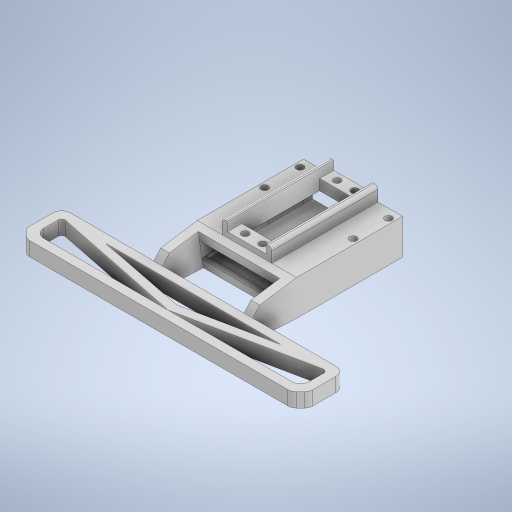
# Autodesk Inventor part: Pieza2
Saved by Autodesk Inventor 2024.3 (Build 283343000, 343)
## iProperties
Created: 2025-01-30
Part Number: Pieza2
Material: Genérico
Document SubType Name: Modeling
Designer: Jorge
Density: 1 g/cm^3
Appearance: Valor por defecto
Author: Jorge
Autodesk Inventor part; units mm, degrees
sketch "Boceto1" plane through (0, 0, 0) normal (0, 1, 0) x (-1, 0, 0)
  line L0 (0, 0) -> (0, -60)
  line L1 (0, 0) -> (30, 0)
  line L2 (0, -60) -> (30, -60)
  line L3 (30, -60) -> (30, 0)
  line L4 (0, 0) -> (-26, 0)
  line L5 (-26, 0) -> (-26, -60)
  line L6 (-26, -60) -> (0, -60)
  dimension "d0" = 60
  dimension "d1" = 30
  dimension "d2" = 30
  dimension "d3" = 26
  constraints: 14 end point, 3 horizontal, 1 collinear, 1 perpendicular, 1 vertical
  measures "d0" distance of L0.start L0.end
  measures "d1" distance of L0.start L1.end
  measures "d2" distance of L0.end L2.end
  measures "d3" distance of L0.start L4.end
extrude "Extrusión1" add sketch "Boceto1" along normal blind 20
sketch "Boceto2" plane through (-30, 0, 0) normal (0, 0, 1) x (1, 0, 0)
  line L0 (56, 0) -> (0, 0) construction
  line L1 (28, 0) -> (28, 20) construction
  line L2 (56, 20) -> (0, 20) construction
  line L3 (0, 0) -> (0, 20) construction
  line L4 (0, 10) -> (5, 10) construction
  line L5 (56, 0) -> (56, 20) construction
  line L6 (56, 10) -> (51, 10) construction
  line L7 (28, 20) -> (28, 17) construction
  line L8 (28, 17) -> (51, 17)
  line L9 (51, 17) -> (51, 10)
  line L10 (28, 17) -> (5, 17)
  line L11 (5, 17) -> (5, 10)
  line L12 (28, 0) -> (28, 3) construction
  line L13 (28, 3) -> (5, 3)
  line L14 (5, 3) -> (5, 10)
  line L15 (28, 3) -> (51, 3)
  line L16 (51, 3) -> (51, 10)
  point P0 (30, 0)
  dimension "d8" = 3
  dimension "d9" = 3
  constraints: 26 end point, 5 perpendicular, 4 midpoint, 4 point on line, 2 horizontal, 1 collinear
  measures "d8" distance of L1.end L7.end
  measures "d9" distance of L1.start L12.end
extrude "Extrusión2" cut sketch "Boceto2" against normal through all
sketch "Boceto3" plane through (0, 20, 0) normal (0, 1, 0) x (1, 0, 0)
  line L0 (21, 60) -> (-25, 60) projected
  line L1 (-2, 60) -> (-2, 0)
  line L2 (-25, 0) -> (21, 0) projected
  line L3 (-2, 0) -> (12, 0) construction
  line L4 (-2, 0) -> (-16, 0) construction
  line L5 (-16, 0) -> (-16, 60) construction
  line L6 (-16, 60) -> (12, 60)
  line L7 (12, 60) -> (12, 0)
  line L8 (12, 0) -> (-16, 0)
  line L9 (-16, 0) -> (-16, 60)
  point P0 (0, 0)
  point P1 (12, 60)
  dimension "d12" = 14
  dimension "d13" = 14
  constraints: 16 end point, 3 point on line, 2 midpoint, 2 parallel, 2 perpendicular, 1 horizontal
  measures "d12" distance of L1.end L3.end
  measures "d13" distance of L1.end L4.end
extrude "Extrusión3" add sketch "Boceto3" along normal blind 8
sketch "Boceto4" plane through (0, 28, 0) normal (0, 1, 0) x (1, 0, 0)
  line L0 (12, 0) -> (26, 0) construction
  line L1 (12, 0) -> (9, 0) construction
  line L2 (9, 0) -> (9, 60)
  line L3 (26, 60) -> (-30, 60) projected
  line L4 (-16, 0) -> (-16, 60) projected
  line L5 (-16, 0) -> (-13, 0)
  line L6 (-30, 0) -> (26, 0) projected
  line L7 (-13, 0) -> (-13, 60)
  line L8 (-2, 0) -> (-2, 8) construction
  line L9 (-13, 8) -> (9, 8)
  line L10 (-2, 60) -> (-2, 52) construction
  line L11 (-13, 52) -> (9, 52)
  line L12 (9, 56) -> (5, 56) construction
  line L13 (-13, 30) -> (9, 30) construction
  line L14 (5, 56) -> (3, 56) construction
  circle A0 centre (3, 56) radius 2
  circle A1 centre (-7, 56) radius 2
  circle A2 centre (3, 4) radius 2
  circle A3 centre (-7, 4) radius 2
  point P0 (0, 0)
  dimension "d16" = 3
  dimension "d17" = 3
  dimension "d18" = 8
  dimension "d19" = 8
  dimension "d20" = 4
  dimension "d21" = 2
  constraints: 22 end point, 8 point on line, 4 midpoint, 3 centre point, 3 horizontal, 3 perpendicular, 3 symmetric about line, 3 vertical, 1 coincident, 1 horizontal alignment, 5 other
  measures "d16" distance of L0.start L1.end
  measures "d17" distance of L4.start L5.end
  measures "d18" distance of L8.start L8.end
  measures "d19" distance of L10.start L10.end
  measures "d20" distance of L12.start L12.end
  measures "d21" distance of L12.end L14.end
extrude "Extrusión4" cut sketch "Boceto4" against normal blind 15 contours L9 L7 L11 L2
extrude "Extrusión5" cut sketch "Boceto4" against normal blind 15 contours A0 | A1 | A2 | A3
extrude "Extrusión6" cut sketch "Boceto4" against normal blind 5 contours L6 L7 L9 L2 | L11 L7 L3 L2
fillet "Empalme1" radius 2 2 edges at (-16, 28, -30) (12, 28, -30)
ref_plane "Plano de trabajo1" through (-2, 0, 0) normal (1, 0, 0) x (0, 1, 0)
sketch "Boceto6" plane through (-2, 0, 0) normal (1, 0, 0) x (0, 1, 0)
  line L0 (0, 0) -> (20, 0) projected
  line L1 (28, 0) -> (23, 0) projected
  line L2 (28, 0) -> (0, 0)
  line L3 (20, 0) -> (16.2743, 24.7208)
  line L4 (16.2743, 24.7208) -> (1.2743, 24.7208)
  line L5 (1.2743, 24.7208) -> (0, 0)
  line L6 (0, 0) -> (20, 0)
  dimension "d32" = 25
  dimension "d33" = 15
  constraints: 10 end point, 2 horizontal, 1 collinear
  measures "d32" distance of L0.end L3.end
  measures "d33" distance of L3.end L4.end
extrude "Extrusión7" add sketch "Boceto6" along normal mid plane 56
sketch "Boceto7" plane through (-30, 16.2743, 24.7208) normal (0, 0.9888, 0.149) x (1, 0, 0)
  line L0 (56, -2.2354) -> (56, 22.0194) construction
  line L1 (56, 9.892) -> (51, 9.892) construction
  line L2 (0, 22.0194) -> (0, -2.2354) construction
  line L3 (0, 11.3809) -> (5, 11.3809) construction
  line L4 (39, 25.4471) -> (17, 25.4471) construction
  line L5 (28, 25.4471) -> (28, 20.4471) construction
  line L6 (0, 0) -> (56, 0) projected
  line L7 (5, 0) -> (51, 0)
  line L8 (51, 0) -> (51, 20.4471)
  line L9 (51, 20.4471) -> (5, 20.4471)
  line L10 (5, 20.4471) -> (5, 0)
  line L11 (5, 0) -> (5, -22.0119)
  line L12 (5, -22.0119) -> (51, -22.0119)
  line L13 (51, -22.0119) -> (51, 0)
  point P0 (30, 22.0194)
  dimension "d36" = 5
  dimension "d38" = 5
  dimension "d39" = 5
  constraints: 20 end point, 3 horizontal, 2 midpoint, 2 parallel, 2 perpendicular, 2 point on line, 2 vertical, 1 collinear
  measures "d36" distance of L1.start L1.end
  measures "d38" distance of L3.start L3.end
  measures "d39" distance of L5.start L5.end
extrude "Extrusión8" cut sketch "Boceto7" against normal blind 56
ref_plane "Plano de trabajo2" through (26, 0, 24.73) normal (0, 0, -1) x (-1, 0, 0)
sketch "Boceto8" plane through (26, 0, 24.73) normal (0, 0, -1) x (-1, 0, 0)
  line L0 (17, 23) -> (39, 23) construction
  line L1 (28, 23) -> (28, 0) construction
  line L2 (56, 0) -> (0, 0) construction
  line L3 (28, 8.5182) -> (108, 8.5182) construction
  line L4 (28, 8.5182) -> (-52, 8.5182) construction
  line L5 (28, 8.5182) -> (28, 12.5182) construction
  line L6 (28, 8.5182) -> (28, 4.5182) construction
  line L7 (-52, 12.5182) -> (108, 12.5182)
  line L8 (108, 12.5182) -> (108, 4.5182)
  line L9 (108, 4.5182) -> (-52, 4.5182)
  line L10 (-52, 4.5182) -> (-52, 12.5182)
  point P0 (26, 0)
  dimension "d43" = 80
  dimension "d44" = 80
  dimension "d45" = 4
  dimension "d46" = 4
  constraints: 18 end point, 3 point on line, 2 horizontal, 2 midpoint, 2 parallel, 2 perpendicular
  measures "d43" distance of L3.start L3.end
  measures "d44" distance of L3.start L4.end
  measures "d45" distance of L3.start L5.end
  measures "d46" distance of L3.start L6.end
extrude "Extrusión9" add sketch "Boceto8" against normal blind 25
fillet "Empalme2" radius 5 2 edges at (78, 8.5182, 24.73) (-82, 8.5182, 24.73)
sketch "Boceto9" plane through (-82, 12.5182, 49.73) normal (0, 1, 0) x (1, 0, 0)
  line L0 (0, 0) -> (160, 0) construction
  line L1 (0, 0) -> (0, 5) construction
  line L2 (0, 20) -> (0, 0) construction
  line L3 (0, 5) -> (5, 5) construction
  line L4 (5, 5) -> (5, 0) construction
  line L5 (160, 20) -> (160, 0) construction
  line L6 (160, 0) -> (160, 5) construction
  line L7 (160, 5) -> (155, 5) construction
  line L8 (155, 5) -> (155, 0) construction
  line L9 (5, 0) -> (0, 5)
  line L10 (155, 0) -> (160, 5)
  line L11 (5, 0) -> (0, 0)
  line L12 (0, 0) -> (0, 5)
  line L13 (155, 0) -> (160, 0)
  line L14 (160, 0) -> (160, 5)
  point P0 (82, 49.73)
  dimension "d50" = 5
  dimension "d51" = 5
  dimension "d52" = 5
  dimension "d53" = 5
  constraints: 24 end point, 6 perpendicular, 3 point on line, 1 collinear
  measures "d50" distance of L0.start L1.end
  measures "d51" distance of L1.end L3.end
  measures "d52" distance of L0.end L6.end
  measures "d53" distance of L6.end L7.end
extrude "Extrusión10" cut sketch "Boceto9" against normal through all
fillet "Empalme3" radius 5 4 edges at (-82, 8.5182, 44.73) (78, 8.5182, 44.73) (73, 8.5182, 49.73) (-77, 8.5182, 49.73)
sketch "Boceto10" plane through (-77, 12.5182, 24.73) normal (0, 1, 0) x (1, 0, 0)
  line L0 (150, 0) -> (0, 0) construction
  line L1 (75, 0) -> (75, -5) construction
  line L2 (2.0711, -25) -> (147.9289, -25) construction
  line L3 (75, -25) -> (75, -20) construction
  line L4 (-5, -5) -> (-5, -17.9289) construction
  line L5 (-5, -11.4645) -> (0, -11.4645) construction
  line L6 (155, -5) -> (155, -17.9289) construction
  line L7 (155, -11.4645) -> (150, -11.4645) construction
  line L8 (2, -5) -> (148, -5)
  line L9 (150, -7) -> (150, -15)
  line L10 (145, -20) -> (5, -20)
  line L11 (0, -15) -> (0, -7)
  arc A0 (2, -5) -> (0, -7) centre (2, -7) ccw
  arc A1 (150, -7) -> (148, -5) centre (148, -7) ccw
  arc A2 (0, -15) -> (5, -20) centre (5, -15) ccw
  arc A3 (145, -20) -> (150, -15) centre (145, -15) ccw
  point P0 (77, 24.73)
  dimension "d57" = 5
  dimension "d58" = 5
  dimension "d59" = 5
  dimension "d60" = 2
  dimension "d61" = 2
  dimension "d62" = 5
  constraints: 16 end point, 8 point on circle, 8 tangent, 4 centre point, 4 midpoint, 3 horizontal, 2 parallel, 2 vertical, 1 equal radius, 1 perpendicular
  measures "d57" distance of L1.start L1.end
  measures "d58" distance of L3.start L3.end
  measures "d59" distance of L7.start L7.end
  measures "d60" radius of A0
  measures "d61" radius of A1
  measures "d62" radius of A2
extrude "Extrusión11" cut sketch "Boceto10" against normal through all
ref_plane "Plano de trabajo3" through (-77, 12.5182, 24.73) normal (0, 1, 0) x (1, 0, 0)
sketch "Boceto11" plane through (-77, 12.5182, 24.73) normal (0, 1, 0) x (1, 0, 0)
  line L0 (2, -5) -> (148, -5) projected
  line L1 (2, -5) -> (75, -20)
  line L2 (145, -20) -> (5, -20) projected
  line L3 (148, -5) -> (75, -20)
  line L4 (75, -20) -> (75, -15) construction
  line L5 (75, -20) -> (80, -20) construction
  line L6 (75, -15) -> (123.6667, -5)
  line L7 (75, -15) -> (25.1063, -5)
  line L8 (2, -5) -> (25.1063, -5)
  line L9 (123.6667, -5) -> (148, -5)
  point P0 (77, 24.73)
  dimension "d67" = 5
  dimension "d68" = 90
  constraints: 16 end point, 2 collinear, 2 point on line, 1 horizontal, 1 midpoint, 1 perpendicular, 1 vertical
  measures "d67" distance of L1.end L4.end
  measures "d68" angle of L5 L4
extrude "Extrusión12" add sketch "Boceto11" against normal blind 8 contours L0 L7 L6 L3 L1
chamfer "Chaflán1" distance 4 angle 45 4 edges at (23.5, 1.2743, 24.7208) (-27.5, 1.2743, 24.7208) (23.5, 16.2743, 24.7208) (-27.5, 16.2743, 24.7208)
sketch "Boceto12" plane through (0, 0, 0) normal (0, -1, 0) x (1, 0, 0)
  line L0 (26, -60) -> (-30, -60) construction
  line L1 (-25, 0) -> (-25, -60) construction
  line L2 (-30, -60) -> (-25, -60) construction
  line L3 (-27.5, -60) -> (-27.5, -55) construction
  line L4 (-30, -60) -> (-30, 0) construction
  line L5 (-30, -55) -> (-25, -55) construction
  line L6 (-25, -55) -> (-27, -55) construction
  circle A0 centre (-27, -55) radius 2
  line L7 (-2, -60) -> (-2, 0) construction
  circle A1 centre (23, -55) radius 2
  line L8 (26, -60) -> (26, -30) construction
  line L9 (26, 0) -> (26, -60) construction
  line L10 (26, -30) -> (-30, -30) construction
  line L11 (-30, -30.4996) -> (-30, -45.4996) construction
  line L12 (-30, -45.4996) -> (26, -45.4996) construction
  line L13 (-27, -55) -> (-27, -35) construction
  circle A2 centre (-27, -35) radius 2
  line L14 (23, -55) -> (23, -35) construction
  circle A3 centre (23, -35) radius 2
  point P0 (0, 0)
  dimension "d74" = 5
  dimension "d79" = 2
  dimension "d80" = 4
  dimension "d81" = 30
  dimension "d82" = 15
  dimension "d83" = 20
  dimension "d84" = 4
  dimension "d85" = 20
  dimension "d86" = 4
  constraints: 22 end point, 6 point on line, 4 centre point, 4 coincident, 4 midpoint, 4 perpendicular, 3 vertical, 1 symmetric about line, 1 other
  measures "d74" distance of L3.start L3.end
  measures "d79" distance of L6.start L6.end
  measures "d80" diameter of A0
  measures "d81" distance of L0.start L8.end
  measures "d82" distance of L11.start L11.end
  measures "d83" distance of L13.start L13.end
  measures "d84" diameter of A2
  measures "d85" distance of L14.start L14.end
  measures "d86" diameter of A3
extrude "Extrusión13" cut sketch "Boceto12" against normal through all
sketch "Boceto13" plane through (-25, 19.3215, 4.5021) normal (0, -0.149, 0.9888) x (1, 0, 0)
  line L0 (9, 0) -> (37, 0) construction
  line L1 (23, 0) -> (23, -5) construction
  line L2 (-5, -5) -> (51, -5)
  line L3 (51, -5) -> (51, -14.777)
  line L4 (51, -14.777) -> (-5, -14.777)
  line L5 (-5, -14.777) -> (-5, -5)
  line L6 (46, -25.7518) -> (46, -11.9082) projected
  line L7 (46, -14.777) -> (46, -5)
  line L8 (46, -2.9665) -> (46, -16.8102) projected
  line L9 (-0.2144, -14.777) -> (-0.2144, -5)
  point P0 (25, -19.7767)
  dimension "d87" = 5
  dimension "d88" = 9.777
  constraints: 14 end point, 6 point on line, 2 parallel, 2 perpendicular, 1 horizontal, 1 midpoint, 1 vertical
  measures "d87" distance of L1.start L1.end
  measures "d88" distance of L2.end L3.end
extrude "Extrusión14" cut sketch "Boceto13" against normal blind 10 contours L2 L7 L6 L4 L9
